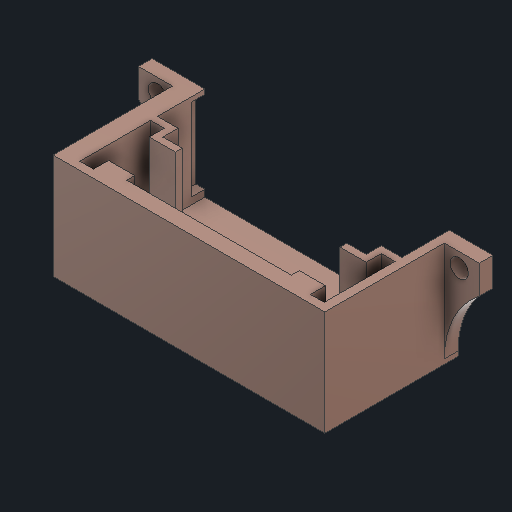
# Autodesk Inventor part: Guía
Saved by Autodesk Inventor 2026 (Build 300175000, 175)
## iProperties
Created: 2025-08-24
Part Number: Guía
Material: Plástico PC/ABS
Document SubType Name: Modeling
Designer: Thomas
Density: 1.1 g/cm^3
Appearance: Suave - Blanco
Author: Thomas
Autodesk Inventor part; units mm, degrees
ref_plane "YZ Plane" through (0, 0, 0) normal (1, 0, 0) x (0, 1, 0)
ref_plane "XZ Plane" through (0, 0, 0) normal (0, 1, 0) x (-1, 0, 0)
ref_plane "XY Plane" through (0, 0, 0) normal (0, 0, 1) x (1, 0, 0)
sketch "Boceto1" plane through (0, 0, 0) normal (0, 1, 0) x (-1, 0, 0)
  line L0 (24, 13.57) -> (26.5, 13.57)
  line L1 (-26.5, 13.57) -> (26.5, -13.57) construction
  line L2 (26.5, 13.57) -> (-26.5, -13.57) construction
  line L3 (24, 13.57) -> (24, 10.27) construction
  line L4 (24, 10.27) -> (20, 10.27) construction
  line L5 (20, 10.27) -> (20, 1.87) construction
  line L6 (20, 1.87) -> (24, 1.87) construction
  line L7 (24, 1.87) -> (24, -1.43) construction
  line L8 (24, -1.43) -> (26.5, -1.43) construction
  line L9 (26.75, -1.68) -> (23.75, -1.68)
  line L10 (23.75, -1.68) -> (23.75, 1.62)
  line L11 (23.75, 1.62) -> (19.5, 1.62)
  line L12 (19.5, 10.52) -> (23.75, 10.52)
  line L13 (23.75, 10.52) -> (23.75, 13.82)
  line L14 (27, 15.57) -> (0, 15.57)
  line L15 (18, 0.12) -> (22.25, 0.12)
  line L16 (22.25, 0.12) -> (22.25, -3.18)
  line L17 (22.25, -3.18) -> (26.75, -3.18)
  line L18 (18, 12.27) -> (0, 12.27)
  line L19 (19.5, 10.52) -> (18, 10.52)
  line L20 (19.5, 1.62) -> (18, 1.62)
  line L21 (27, 15.57) -> (29.75, 15.57)
  line L22 (29.75, 15.57) -> (29.75, -10.57)
  line L23 (29.75, -10.57) -> (36.3, -10.57)
  line L24 (36.3, -10.57) -> (36.3, -13.57)
  line L25 (36.3, -13.57) -> (26.75, -13.57)
  line L26 (0, 12.27) -> (0, 15.57)
  line L27 (23.75, 13.82) -> (26.75, 13.82)
  line L28 (18, 12.27) -> (18, 10.52)
  line L29 (18, 1.62) -> (18, 0.12)
  line L30 (26.75, -13.57) -> (26.75, -3.18)
  line L31 (26.75, -1.68) -> (26.75, 13.82)
  line L32 (26.5, 13.57) -> (26.5, -1.68) construction
  point P0 (0, 0)
  point P1 (23.75, 13.57)
  point P2 (0, 13.57)
  point P3 (27, -12.07)
  dimension "d1" = 27.14
  dimension "d2" = 15
  dimension "d4" = 3.3
  dimension "d5" = 4
  dimension "d6" = 3.3
  dimension "d10" = 0.25
  dimension "d11" = 0.25
  dimension "d12" = 1.5
  dimension "d16" = 3
  dimension "d17" = 29.14
  dimension "d23" = 18
  dimension "d24" = 2
  dimension "d25" = 0.25
  dimension "d27" = 15.57
  dimension "d28" = 29.75
  dimension "d29" = 3.3
  dimension "d30" = 0.25
  dimension "d31" = 20
  dimension "d32" = 6.5
  dimension "d33" = 0.25
  dimension "d34" = 4.25
  dimension "d36" = 0.25
  dimension "d51" = 36.3
  constraints: 66 end point, 16 perpendicular, 6 horizontal, 4 point on line, 2 midpoint, 2 vertical, 2 vertical alignment, 3 other
  measures "d1" distance of L0.end L1.end
  measures "d2" distance between parallel lines of L0 L8
  measures "d4" distance of L0.start L3.end
  measures "d5" distance of L3.end L4.end
  measures "d6" distance of L6.end L7.end
  measures "d10" distance between parallel lines of L9 L8
  measures "d11" distance between parallel lines of L3 L13
  measures "d12" distance between parallel lines of L11 L15
  measures "d16" distance of L23.end L24.end
  measures "d17" distance between parallel lines of L25 L21
  measures "d23" distance of L18.start L18.end
  measures "d24" distance between parallel lines of L14 L0
  measures "d25" distance between parallel lines of L0 L27
  measures "d27" distance from line of L14 point (0, 0)
  measures "d28" distance from line of L14.end L22
  measures "d29" distance of L18.end L14.end
  measures "d30" distance between parallel lines of L4 L12
  measures "d31" distance from line of point (0, 0) L5
  measures "d32" distance between parallel lines of L32 L5
  measures "d33" distance between parallel lines of L10 L7
  measures "d34" distance of L15.start L15.end
  measures "d36" distance between parallel lines of L31 L32
  measures "d51" distance from line of L24 point (0, 0)
extrude "Extrusión1" add sketch "Boceto1" along normal blind 20
mirror "Simetría1" about plane through (0, 0, 0) normal (1, 0, 0) of "Extrusión1"
sketch "Boceto2" plane through (0, 0, 0) normal (0, -1, 0) x (1, 0, 0)
  line L0 (18, 1.62) -> (18, 0.12) projected
  line L1 (18, 1.62) -> (-18, 1.62)
  line L2 (-18, 1.62) -> (-18, 0.12) projected
  line L3 (-18, 0.12) -> (-22.25, 0.12) projected
  line L4 (-22.25, 0.12) -> (-22.25, -3.18) projected
  line L5 (-22.25, -3.18) -> (-26.75, -3.18) projected
  line L6 (-26.75, -3.18) -> (-26.75, -13.57) projected
  line L7 (26.75, -3.18) -> (26.75, -13.57) projected
  line L8 (22.25, -3.18) -> (26.75, -3.18) projected
  line L9 (22.25, 0.12) -> (22.25, -3.18) projected
  line L10 (18, 0.12) -> (22.25, 0.12) projected
  line L11 (26.75, -13.57) -> (36.3, -13.57) projected
  line L12 (36.3, -13.57) -> (36.3, -10.57) projected
  line L13 (-36.3, -10.57) -> (-29.75, -10.57) projected
  line L14 (-36.3, -13.57) -> (-36.3, -10.57) projected
  line L15 (-26.75, -13.57) -> (-36.3, -13.57) projected
  line L16 (23.75, 1.62) -> (18, 1.62) projected
  line L17 (23.75, -1.68) -> (23.75, 1.62) projected
  line L18 (26.75, -1.68) -> (23.75, -1.68) projected
  line L19 (36.3, -10.57) -> (29.75, -10.57) projected
  line L20 (26.75, -1.68) -> (29.75, -1.68)
  line L21 (29.75, -10.57) -> (29.75, 15.57) projected
  line L22 (-23.75, 1.62) -> (-18, 1.62) projected
  line L23 (-23.75, -1.68) -> (-23.75, 1.62) projected
  line L24 (-26.75, -1.68) -> (-23.75, -1.68) projected
  line L25 (-26.75, 13.82) -> (-26.75, -1.68) projected
  line L26 (-26.75, -1.68) -> (-29.75, -1.68)
  line L27 (-29.75, -10.57) -> (-29.75, 15.57) projected
  line L28 (26.75, -13.57) -> (-26.75, -13.57)
  line L29 (-18, 12.27) -> (18, 12.27) projected
  line L30 (12.75, 12.27) -> (12.75, 1.62)
  line L31 (26.75, 13.82) -> (26.75, -1.68) projected
  line L32 (-29.75, 15.57) -> (29.75, 15.57) projected
  line L33 (-16.75, 12.27) -> (-16.75, 1.62)
  line L34 (23.75, 13.82) -> (26.75, 13.82) projected
  line L35 (18, 10.52) -> (23.75, 10.52) projected
  line L36 (23.75, 10.52) -> (23.75, 13.82) projected
  line L37 (18, 12.27) -> (18, 10.52) projected
  line L38 (-23.75, 10.52) -> (-23.75, 13.82) projected
  line L39 (-18, 10.52) -> (-23.75, 10.52) projected
  line L40 (-18, 12.27) -> (-18, 10.52) projected
  line L41 (-18, 12.27) -> (18, 12.27) projected
  line L42 (18, 12.27) -> (18, 10.52) projected
  line L43 (18, 10.52) -> (23.75, 10.52) projected
  line L44 (23.75, 10.52) -> (23.75, 13.82) projected
  line L45 (23.75, 13.82) -> (26.75, 13.82) projected
  line L46 (26.75, 13.82) -> (26.75, -1.68) projected
  line L47 (26.75, -1.68) -> (23.75, -1.68) projected
  line L48 (23.75, -1.68) -> (23.75, 1.62) projected
  line L49 (23.75, 1.62) -> (18, 1.62) projected
  line L50 (18, 1.62) -> (18, 0.12) projected
  line L51 (18, 0.12) -> (22.25, 0.12) projected
  line L52 (22.25, 0.12) -> (22.25, -3.18) projected
  line L53 (22.25, -3.18) -> (26.75, -3.18) projected
  line L54 (26.75, -3.18) -> (26.75, -13.57) projected
  line L55 (26.75, -13.57) -> (36.3, -13.57) projected
  line L56 (36.3, -13.57) -> (36.3, -10.57) projected
  line L57 (36.3, -10.57) -> (29.75, -10.57) projected
  line L58 (29.75, -10.57) -> (29.75, 15.57) projected
  line L59 (-29.75, 15.57) -> (29.75, 15.57) projected
  line L60 (-29.75, -10.57) -> (-29.75, 15.57) projected
  line L61 (-36.3, -10.57) -> (-29.75, -10.57) projected
  line L62 (-36.3, -13.57) -> (-36.3, -10.57) projected
  line L63 (-26.75, -13.57) -> (-36.3, -13.57) projected
  line L64 (-26.75, -3.18) -> (-26.75, -13.57) projected
  line L65 (-22.25, -3.18) -> (-26.75, -3.18) projected
  line L66 (-22.25, 0.12) -> (-22.25, -3.18) projected
  line L67 (-18, 0.12) -> (-22.25, 0.12) projected
  line L68 (-18, 1.62) -> (-18, 0.12) projected
  line L69 (-23.75, 1.62) -> (-18, 1.62) projected
  line L70 (-23.75, -1.68) -> (-23.75, 1.62) projected
  line L71 (-26.75, -1.68) -> (-23.75, -1.68) projected
  line L72 (-26.75, 13.82) -> (-26.75, -1.68) projected
  line L73 (-23.75, 13.82) -> (-26.75, 13.82) projected
  line L74 (18, 10.52) -> (12.75, 10.52)
  line L75 (-18, 10.52) -> (-16.75, 10.52)
  point P0 (0, 0)
  point P1 (0, 1.62)
  point P2 (12.75, 12.27)
  dimension "d42" = 14
  dimension "d43" = 10
  constraints: 16 end point, 8 point on line, 2 horizontal, 2 perpendicular, 1 collinear, 1 midpoint
  measures "d42" distance between parallel lines of L31 L30
  measures "d43" distance between parallel lines of L25 L33
extrude "Extrusión2" add sketch "Boceto2" along normal blind 3 contours L16 L17 L18 L20 L21 L19 L12 L11 L7 L8 L9 L10 L0 | L0 L10 L9 L8 L7 L28 L6 L5 L4 L3 L2 L1 | L1 L33 L29 L30 | L30 L29 L37 L74 | L2 L3 L4 L5 L6 L15 L14 L13 L27 L26 L24 L23 L22 | L75 L40 L29 L33 | L29 L40 L39 L38 L73 L25 L26 L27 L32 L21 L20 L31 L34 L36 L35 L37
move faces "Desplazar2" translate (0, -0.5, 0) faces at (4.25, 0, -8.5067)
move faces "Desplazar3" translate (-1.1, 0, 0) faces at (-29.75, 12.3333, 6.8567)
move faces "Desplazar4" translate (-1.1, 0, 0) faces at (29.75, 12.3333, 6.8567)
move faces "Desplazar5" translate (-2, 0, 0) faces at (-36.3, 12.3333, -11.57)
sketch "Boceto5" plane through (-36.3, -3, -10.57) normal (0, 0, 1) x (1, 0, 0)
  line L0 (0, 0) -> (72.6, 0) projected
  line L1 (5.45, 0) -> (5.45, 23) projected
  line L2 (0, 0) -> (5.45, 0)
  line L3 (5.45, 0) -> (5.45, 16.75)
  line L4 (5.45, 16.75) -> (-2, 16.75)
  line L5 (-2, 16.75) -> (-2, 0)
  line L6 (64.95, 23) -> (64.95, 0) projected
  line L7 (64.95, 0) -> (72.6, 0)
  line L8 (72.6, 0) -> (72.6, 16.75)
  line L9 (72.6, 16.75) -> (64.95, 16.75)
  line L10 (64.95, 16.75) -> (64.95, 0)
  line L11 (72.6, 23) -> (64.95, 23) projected
  line L12 (5.45, 0) -> (-2, 0) projected
  point P0 (36.3, 3)
  dimension "d63" = 6.25
  constraints: 16 end point, 4 parallel, 2 horizontal, 2 perpendicular, 2 point on line, 1 coincident
  measures "d63" distance between parallel lines of L9 L11
extrude "Extrusión5" cut sketch "Boceto5" against normal blind 10
fillet "Empalme2" radius 20 2 edges at (28.65, 13.75, -12.07) (-30.85, 13.75, -12.07)
sketch "Boceto7" plane through (36.3, 20, -13.57) normal (0, 0, -1) x (-1, 0, 0)
  line L0 (65.05, -19) -> (63.05, -19)
  line L1 (63.05, -19) -> (63.05, -1)
  line L2 (63.05, -1) -> (65.05, -1)
  line L3 (65.05, -1) -> (65.05, -19)
  line L4 (63.05, -20.5) -> (9.55, -20.5) projected
  line L5 (63.05, -20.5) -> (63.05, 0) projected
  point P0 (36.3, -20)
  dimension "d75" = 2
  dimension "d76" = 18
  dimension "d77" = 1.5
  constraints: 8 end point, 2 parallel, 1 collinear, 1 horizontal, 1 perpendicular
  measures "d75" distance of L1.end L2.end
  measures "d76" distance of L0.end L1.end
  measures "d77" distance between parallel lines of L0 L4
extrude "Extrusión7" cut sketch "Boceto7" against normal blind 3
sketch "Boceto8" plane through (-38.3, 20, -10.57) normal (0, 0, 1) x (1, 0, 0)
  circle A0 centre (4.175, -3.125) radius 2 projected
  circle A1 centre (70.225, -3.125) radius 2 projected
  circle A2 centre (4.175, -3.125) radius 3
  circle A3 centre (70.225, -3.125) radius 3
  point P0 (38.3, -20)
  dimension "d80" = 6
  dimension "d81" = 6
  constraints: 2 centre point, 2 coincident
  measures "d80" diameter of A2
  measures "d81" diameter of A3
extrude "Extrusión8" cut sketch "Boceto8" against normal through all contours A0 | A1
equation "\"d6\" = d4"
equation "\"d9\" = d7"
equation "\"d7\" = 0.5"
